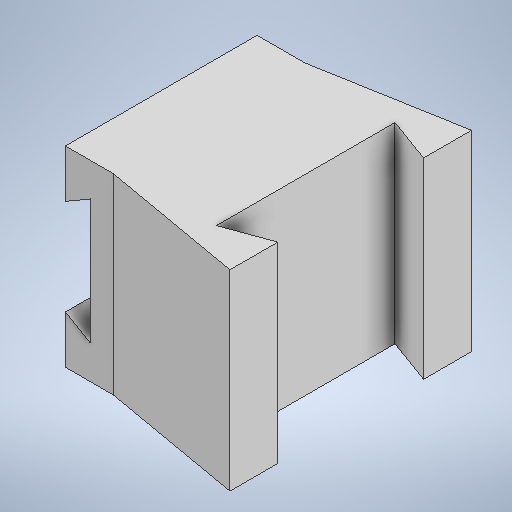
# Autodesk Inventor part: Part1x
Saved by Autodesk Inventor 2025.2 (Build 292293000, 293)
## iProperties
Created: 2025-04-17
Part Number: Part1x
Material: Generic
Document SubType Name: Sheet Metal
Designer: ziyuz
Density: 1 g/cm^3
Sheet Metal Rule: Default_mm
Appearance: Default
Author: ziyuz
Autodesk Inventor part; units mm, degrees
ref_plane "YZ Plane" through (0, 0, 0) normal (1, 0, 0) x (0, 1, 0)
ref_plane "XZ Plane" through (0, 0, 0) normal (0, 1, 0) x (-1, 0, 0)
ref_plane "XY Plane" through (0, 0, 0) normal (0, 0, 1) x (1, 0, 0)
sketch "Sketch1" plane through (0, 0, 0) normal (0, 1, 0) x (-1, 0, 0)
  line L0 (0, 0) -> (0, -20)
  line L1 (0, -20) -> (-14.7721, -22.6047)
  line L2 (-14.7721, -22.6047) -> (-14.7721, -17.6047)
  line L3 (-14.7721, -17.6047) -> (-10.0737, -19.3148)
  line L4 (0, 0) -> (-14.7721, 2.6047)
  line L5 (-14.7721, 2.6047) -> (-14.7721, -2.3953)
  line L6 (-14.7721, -2.3953) -> (-10.0737, -0.6852)
  line L7 (-10.0737, -0.6852) -> (-10.0737, -19.3148)
  dimension "d0" = 20
  dimension "d1" = 15
  dimension "d2" = 100
  dimension "d3" = 5
  dimension "d4" = 5
  dimension "d5" = 70
  dimension "d6" = 15
  dimension "d7" = 5
  dimension "d8" = 5
  constraints: 16 end point, 2 parallel, 2 vertical
  measures "d0" distance of L0.start L0.end
  measures "d1" distance of L0.end L1.end
  measures "d2" angle of L0 L1
  measures "d3" distance of L1.end L2.end
  measures "d4" distance of L2.end L3.end
  measures "d5" angle of L2 L3
  measures "d6" distance of L0.start L4.end
  measures "d7" distance of L4.end L5.end
  measures "d8" distance of L5.end L6.end
extrude "Extrusion1" add sketch "Sketch1" along normal blind 20
sketch "Sketch2" plane through (0, 0, -20) normal (-1, 0, 0) x (0, 0, 1)
  line L0 (0, 0) -> (0, 20) projected
  line L1 (20, 0) -> (0, 0)
  line L2 (0, 0) -> (0, 20)
  line L3 (0, 20) -> (20, 20)
  line L4 (20, 20) -> (20, 0)
  constraints: 8 end point, 2 parallel, 1 horizontal, 1 perpendicular
extrude "Extrusion2" add sketch "Sketch2" along normal blind 5
sketch "Sketch3" plane through (0, 0, -20) normal (0, 0, -1) x (-1, 0, 0)
  line L0 (5, 20) -> (5, 0) projected
  line L1 (5, 20) -> (5, 0)
  line L2 (5, 0) -> (5, 5)
  line L3 (5, 20) -> (5, 15)
  line L4 (5, 15) -> (2.4019, 16.5)
  line L5 (5, 15) -> (8, 15) construction
  line L6 (5, 5) -> (2.4019, 3.5)
  line L7 (2.4019, 3.5) -> (2.4019, 16.5)
  line L8 (5, 20) -> (-5, 20)
  line L9 (5, 15) -> (5, 5)
  point P0 (0, 0)
  point P1 (5, 5)
  dimension "d13" = 5
  dimension "d14" = 5
  dimension "d15" = 3
  dimension "d16" = 150
  dimension "d17" = 3
  constraints: 18 end point, 2 horizontal, 2 point on line, 2 vertical, 1 collinear, 1 equal length
  measures "d13" distance of L0.end L2.end
  measures "d14" distance of L0.start L3.end
  measures "d15" distance of L3.end L4.end
  measures "d16" angle of L5 L4
  measures "d17" distance of L2.end L6.end
extrude "Extrusion3" cut sketch "Sketch3" against normal blind 50
equation "\"BendRadius\" = Thickness"
equation "\"BendReliefWidth\" = Thickness"
equation "\"BendReliefDepth\" = 0.5 * Thickness"
equation "\"CornerReliefSize\" = 4 * Thickness"
equation "\"MinimumRemnant\" = 2 * Thickness"
equation "\"TransitionRadius\" = BendRadius"
equation "\"JacobiRadiusSize\" = BendRadius"
equation "\"GapSize\" = Thickness"
equation "\"Thickness\" = 0.5"
body "Solid1"
